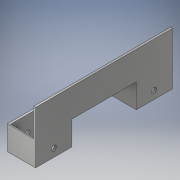
# Autodesk Inventor part: side
Saved by Autodesk Inventor 2016 (Build 200138000, 138)
## iProperties
Created: 2015-10-31
Part Number: side
Material: Generic
Document SubType Name: Modeling
Designer: rossmosier
Density: 1 g/cm^3
Appearance: Aluminum - Polished
Author: rossmosier
Autodesk Inventor part; units mm, degrees
ref_plane "YZ Plane" through (0, 0, 0) normal (1, 0, 0) x (0, 1, 0)
ref_plane "XZ Plane" through (0, 0, 0) normal (0, 1, 0) x (-1, 0, 0)
ref_plane "XY Plane" through (0, 0, 0) normal (0, 0, 1) x (1, 0, 0)
sketch "Sketch1" plane through (0, 0, 0) normal (0, 1, 0) x (-1, 0, 0)
  line L0 (0, 0) -> (-88.9, 0)
  line L1 (-88.9, -114.3) -> (-88.9, -317.5)
  line L2 (-88.9, -431.8) -> (0, -431.8)
  line L3 (0, -431.8) -> (0, 0)
  line L4 (-88.9, 0) -> (-165.1, 0)
  line L5 (-165.1, 0) -> (-165.1, -114.3)
  line L6 (-165.1, -114.3) -> (-88.9, -114.3)
  line L7 (-88.9, -114.3) -> (-88.9, 0)
  line L8 (-88.9, -431.8) -> (-165.1, -431.8)
  line L9 (-165.1, -431.8) -> (-165.1, -317.5)
  line L10 (-165.1, -317.5) -> (-88.9, -317.5)
  line L11 (-88.9, -317.5) -> (-88.9, -431.8)
  line L12 (-88.9, -374.65) -> (-139.7, -374.65) construction
  line L13 (-88.9, -58.8342) -> (-139.7, -58.8342) construction
  circle A0 centre (-139.7, -58.8342) radius 7.9375
  circle A1 centre (-139.7, -374.65) radius 7.9375
  dimension "d0" = 88.9
  dimension "d1" = 431.8
  dimension "d2" = 76.2
  dimension "d3" = 114.3
  dimension "d4" = 76.2
  dimension "d5" = 114.3
  dimension "d6" = 50.8
  dimension "d7" = 15.875
  dimension "d8" = 15.875
  constraints: 28 end point, 6 parallel, 5 horizontal, 3 perpendicular, 2 centre point, 2 coincident, 1 midpoint, 1 point on line
  measures "d0" distance of L2.end L2.start
  measures "d1" distance of L2.start L0.end
  measures "d2" distance of L1.start L5.end
  measures "d3" distance of L5.end L4.end
  measures "d4" distance of L1.end L9.end
  measures "d5" distance of L8.end L9.end
  measures "d6" distance of L12.start L12.end
  measures "d7" diameter of A0
  measures "d8" diameter of A1
extrude "Extrusion1" add sketch "Sketch1" along normal blind 6.35
sketch "Sketch8" plane through (0, 6.35, 0) normal (0, 1, 0) x (1, 0, 0)
  circle A0 centre (139.7, 58.8342) radius 7.9375 projected
  circle A1 centre (139.7, 374.65) radius 7.9375 projected
  line L0 (88.9, 317.5) -> (165.1, 317.5) projected
  line L1 (165.1, 317.5) -> (165.1, 431.8) projected
  line L2 (165.1, 431.8) -> (0, 431.8) projected
  line L3 (0, 431.8) -> (0, 0) projected
  line L4 (0, 0) -> (165.1, 0) projected
  line L5 (165.1, 0) -> (165.1, 114.3) projected
  line L6 (165.1, 114.3) -> (88.9, 114.3) projected
  line L7 (88.9, 114.3) -> (88.9, 317.5) projected
  line L8 (165.1, 0) -> (88.9, 0)
  line L9 (88.9, 0) -> (88.9, 3.175)
  line L10 (88.9, 3.175) -> (165.1, 3.175)
  line L11 (165.1, 3.175) -> (165.1, 0)
  line L12 (165.1, 114.3) -> (88.9, 114.3)
  line L13 (88.9, 114.3) -> (88.9, 111.125)
  line L14 (88.9, 111.125) -> (165.1, 111.125)
  line L15 (165.1, 111.125) -> (165.1, 114.3)
  line L16 (88.9, 114.3) -> (88.9, 317.5) projected
  line L17 (165.1, 317.5) -> (88.9, 317.5)
  line L18 (88.9, 317.5) -> (88.9, 320.675)
  line L19 (88.9, 320.675) -> (165.1, 320.675)
  line L20 (165.1, 320.675) -> (165.1, 317.5)
  line L21 (165.1, 431.8) -> (88.9, 431.8)
  line L22 (88.9, 431.8) -> (88.9, 428.625)
  line L23 (88.9, 428.625) -> (165.1, 428.625)
  line L24 (165.1, 428.625) -> (165.1, 431.8)
  dimension "d27" = 3.175
  dimension "d28" = 3.175
  dimension "d29" = 3.175
  dimension "d30" = 3.175
  constraints: 32 end point, 8 parallel, 4 horizontal, 4 perpendicular, 2 point on line
  measures "d27" distance of L8.end L9.end
  measures "d28" distance of L13.end L12.end
  measures "d29" distance of L17.end L18.end
  measures "d30" distance of L22.end L21.end
extrude "Extrusion7" add sketch "Sketch8" along normal blind 82.55 contours L18 L19 L1 L0 | L6 L5 L14 L13 | L23 L22 L2 L1 | L5 L4 L9 L10
sketch "Sketch9" plane through (165.1, 6.35, -3.175) normal (0, 0, -1) x (-1, 0, 0)
  line L0 (76.2, 0) -> (0, 0) projected
  line L1 (76.2, 0) -> (76.2, 82.55) projected
  line L2 (0, 82.55) -> (76.2, 82.55) projected
  line L3 (0, 0) -> (0, 82.55) projected
  line L4 (0, -6.35) -> (0, 82.55) projected
  line L5 (76.2, 82.55) -> (0, 82.55)
  line L6 (0, 82.55) -> (0, 76.2)
  line L7 (0, 76.2) -> (76.2, 76.2)
  line L8 (76.2, 76.2) -> (76.2, 82.55)
  point P0 (165.1, -6.35)
  dimension "d33" = 6.35
  constraints: 8 end point, 2 parallel, 1 horizontal, 1 perpendicular, 1 point on line
  measures "d33" distance of L6.end L5.end
sketch "Sketch10" plane through (165.1, 6.35, -320.675) normal (0, 0, -1) x (-1, 0, 0)
  line L0 (76.2, -6.35) -> (0, -6.35) projected
  line L1 (0, -6.35) -> (0, 82.55) projected
  line L2 (76.2, 82.55) -> (0, 82.55) projected
  line L3 (76.2, 0) -> (76.2, 82.55) projected
  line L4 (76.2, -6.35) -> (76.2, 0) projected
  line L5 (0, 0) -> (0, 82.55) projected
  line L6 (76.2, 82.55) -> (0, 82.55)
  line L7 (0, 82.55) -> (0, 76.2)
  line L8 (0, 76.2) -> (76.2, 76.2)
  line L9 (76.2, 76.2) -> (76.2, 82.55)
  point P0 (165.1, -6.35)
  dimension "d34" = 6.35
  constraints: 8 end point, 2 parallel, 1 horizontal, 1 perpendicular, 1 point on line
  measures "d34" distance of L7.end L6.end
extrude "Extrusion8" add sketch "Sketch9" along normal blind 107.95 contours L7 L3 L2 L1
extrude "Extrusion9" add sketch "Sketch10" along normal blind 107.95 contours L8 L1 L2 L3
sketch "Sketch11" plane through (88.9, 82.55, -320.675) normal (0, -1, 0) x (1, 0, 0)
  line L0 (0, 0) -> (76.2, 0) projected
  circle A0 centre (50.8, -53.975) radius 7.9375 projected
  line L1 (0, 206.375) -> (0, 3.175) projected
  line L2 (76.2, -111.125) -> (-88.9, -111.125) projected
  line L3 (76.2, 3.175) -> (76.2, -111.125) projected
  line L4 (0, 3.175) -> (76.2, 3.175) projected
  circle A1 centre (50.8, 261.8408) radius 7.9375 projected
  line L5 (0, 206.375) -> (0, 3.175) projected
  line L6 (76.2, 206.375) -> (0, 206.375) projected
  line L7 (76.2, 320.675) -> (76.2, 206.375) projected
  line L8 (-88.9, 320.675) -> (76.2, 320.675) projected
  line L9 (-88.9, -111.125) -> (-88.9, 320.675) projected
  line L10 (76.2, -111.125) -> (-88.9, -111.125) projected
  circle A2 centre (50.8, 261.8408) radius 7.9375 projected
  circle A3 centre (50.8, -53.975) radius 7.9375
  circle A4 centre (50.8, 261.8408) radius 7.9375
  line L11 (76.2, 3.175) -> (76.2, -111.125) projected
  line L12 (0, 3.175) -> (76.2, 3.175) projected
  line L13 (76.2, 206.375) -> (0, 206.375) projected
  line L14 (76.2, 320.675) -> (76.2, 206.375) projected
  line L15 (-88.9, 320.675) -> (76.2, 320.675) projected
  line L16 (-88.9, -111.125) -> (-88.9, 320.675) projected
  constraints: 2 centre point, 2 coincident
extrude "Extrusion10" cut sketch "Sketch11" against normal blind 25.4 contours A0
sketch "Sketch12" plane through (88.9, 82.55, -3.175) normal (0, -1, 0) x (1, 0, 0)
  circle A0 centre (50.8, -55.6592) radius 7.9375 projected
  circle A1 centre (50.8, -55.6592) radius 7.9375
  point P0 (-88.9, 3.175)
  constraints: 1 centre point, 1 coincident, 1 concentric
extrude "Extrusion11" cut sketch "Sketch12" against normal blind 25.4
body "Solid1"
